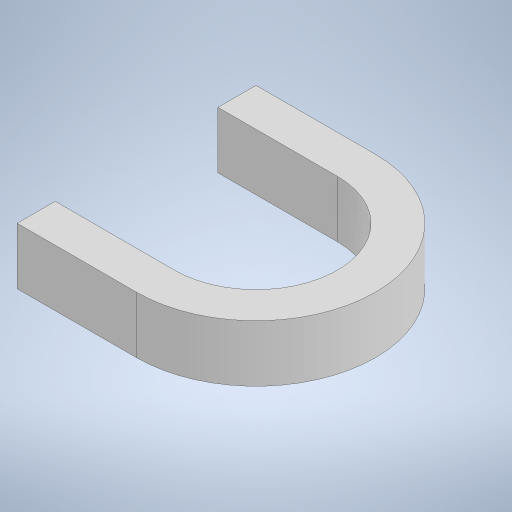
# Autodesk Inventor part: Obrecz_kolanko
Saved by Autodesk Inventor 2024 (Build 280153000, 153)
## iProperties
Created: 2023-12-16
Part Number: Obrecz_kolanko
Material: Generic
Document SubType Name: Modeling
Designer: Piter
Density: 1 g/cm^3
Appearance: Default
Author: Piter
Autodesk Inventor part; units mm, degrees
ref_plane "YZ Plane" through (0, 0, 0) normal (1, 0, 0) x (0, 1, 0)
ref_plane "XZ Plane" through (0, 0, 0) normal (0, 1, 0) x (-1, 0, 0)
ref_plane "XY Plane" through (0, 0, 0) normal (0, 0, 1) x (1, 0, 0)
sketch "Sketch1" plane through (0, 0, 0) normal (0, 1, 0) x (-1, 0, 0)
  circle A0 centre (0, 0) radius 27.25
  circle A1 centre (0, 0) radius 40
  line L0 (0, 40) -> (0, -40)
  line L1 (0, 40) -> (40, 40)
  line L2 (40, 40) -> (40, 27.25)
  line L3 (40, 27.25) -> (0, 27.25)
  line L4 (0, 27.25) -> (0, 40)
  line L5 (0, 0) -> (45.8367, 0)
  line L6 (0, -40) -> (40, -40)
  line L7 (40, -40) -> (40, -27.25)
  line L8 (40, -27.25) -> (0, -27.25)
  line L9 (0, -27.25) -> (0, -40)
  point P0 (0, -27.25)
  point P1 (0, 27.25)
  dimension "d0" = 54.5
  dimension "d1" = 80
  constraints: 20 end point, 3 symmetric about line, 2 centre point, 2 coincident, 2 horizontal, 2 parallel, 2 point on circle, 1 perpendicular, 1 vertical
  measures "d0" diameter of A0
  measures "d1" diameter of A1
extrude "Extrusion1" add sketch "Sketch1" along normal blind 19 contours A0 L0 A1 | L0 A1 L3 | L8 A1 L0 | L1 L2 L3 A1 | A1 L8 L7 L6
body "Solid1"
